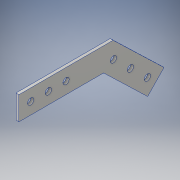
# Autodesk Inventor part: lower gusset
Saved by Autodesk Inventor 2016 (Build 200138000, 138)
## iProperties
Created: 2016-02-23
Part Number: lower gusset
Material: Aluminum 6061
Document SubType Name: Modeling
Designer: gus
Density: 2.7 g/cm^3
Appearance: Aluminum - Flat
Author: gus
Autodesk Inventor part; units mm, degrees
ref_plane "YZ Plane" through (0, 0, 0) normal (1, 0, 0) x (0, 1, 0)
ref_plane "XZ Plane" through (0, 0, 0) normal (0, 1, 0) x (-1, 0, 0)
ref_plane "XY Plane" through (0, 0, 0) normal (0, 0, 1) x (1, 0, 0)
sketch "Sketch1" plane through (0, 0, 0) normal (1, 0, 0) x (0, 1, 0)
  line L0 (0, 0) -> (0, -101.6)
  line L1 (0, -101.6) -> (-52.8555, -156.4884)
  line L2 (-25.4, 2.4125) -> (-25.4, -91.3586)
  line L3 (-25.4, -91.3586) -> (-71.1516, -138.8699)
  line L4 (-52.8555, -156.4884) -> (-71.1516, -138.8699)
  line L5 (0, 0) -> (-25.4, 0)
  dimension "d0" = 101.6
  dimension "d1" = 25.4
  dimension "d2" = 25.4
  dimension "d3" = 76.2
  dimension "d4" = 136.081
  constraints: 12 end point, 2 perpendicular, 2 vertical, 1 parallel, 1 point on line
  measures "d0" distance of L0.start L0.end
  measures "d1" distance between parallel lines of L3 L1
  measures "d2" distance between parallel lines of L2 L0
  measures "d3" distance of L0.end L1.end
  measures "d4" angle of L3 L2
extrude "Extrusion1" add sketch "Sketch1" along normal blind 3.175
sketch "Sketch2" plane through (0, 0, 0) normal (-1, 0, 0) x (0, 0, 1)
  circle A0 centre (-12.7, -12.7) radius 3.3734
  circle A1 centre (-31.75, -12.7) radius 3.3734
  circle A2 centre (-50.8, -12.7) radius 3.3734
  line L0 (0, -25.4) -> (0, 0) projected
  line L1 (0, -12.7) -> (-114.7885, -12.7) construction
  line L2 (-156.4884, -52.8555) -> (-101.6, 0) projected
  circle A3 centre (-138.5311, -53.1943) radius 3.3734
  circle A4 centre (-120.235, -35.5758) radius 3.3734
  circle A5 centre (-101.9388, -17.9573) radius 3.3734
  line L3 (-91.3586, -25.4) -> (-138.8699, -71.1516) projected
  line L4 (-156.4884, -52.8555) -> (-138.8699, -71.1516) projected
  dimension "d7" = 6.7469
  dimension "d8" = 6.7469
  dimension "d9" = 6.7469
  dimension "d10" = 12.7
  dimension "d11" = 19.05
  dimension "d12" = 19.05
  dimension "d15" = 6.7469
  dimension "d16" = 6.7469
  dimension "d17" = 6.7469
  dimension "d18" = 12.7
  dimension "d19" = 12.7
  dimension "d20" = 12.7
  dimension "d21" = 12.7
  dimension "d22" = 38.1
  dimension "d23" = 63.5
  constraints: 6 centre point, 4 point on line, 2 end point, 1 horizontal, 1 midpoint
  measures "d7" diameter of A0
  measures "d8" diameter of A1
  measures "d9" diameter of A2
  measures "d10" distance from line of L0 A0.centre
  measures "d11" distance of A1.centre A0.centre
  measures "d12" distance of A1.centre A2.centre
  measures "d15" diameter of A3
  measures "d16" diameter of A4
  measures "d17" diameter of A5
  measures "d18" distance from line of L3 A4.centre
  measures "d19" distance from line of L3 A5.centre
  measures "d20" distance from line of L3 A3.centre
  measures "d21" distance from line of L4 A3.centre
  measures "d22" distance from line of L4 A4.centre
  measures "d23" distance from line of L4 A5.centre
extrude "Extrusion2" cut sketch "Sketch2" against normal blind 3.175
body "Solid1"
